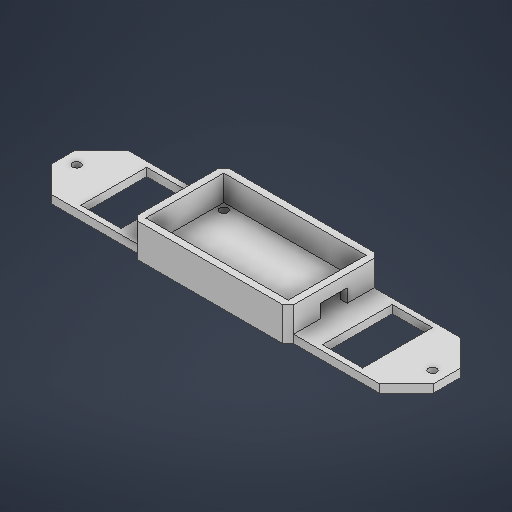
# Autodesk Inventor part: espbase
Saved by Autodesk Inventor 2026 (Build 300175050, 175E)
## iProperties
Created: 2025-04-01
Part Number: espbase
Material: Genérico
Document SubType Name: Modeling
Designer: Ian
Density: 1 g/cm^3
Appearance: Padrão
Author: Ian
Autodesk Inventor part; units mm, degrees
ref_plane "YZ Plane" through (0, 0, 0) normal (1, 0, 0) x (0, 1, 0)
ref_plane "XZ Plane" through (0, 0, 0) normal (0, 1, 0) x (-1, 0, 0)
ref_plane "XY Plane" through (0, 0, 0) normal (0, 0, 1) x (1, 0, 0)
sketch "Esboço1" plane through (0, 0, 0) normal (0, 1, 0) x (-1, 0, 0)
  line L0 (-29, 17) -> (29, 17)
  line L1 (29, 17) -> (29, -17)
  line L2 (29, -17) -> (-29, -17)
  line L3 (-29, -17) -> (-29, 17)
  line L4 (-29, 17) -> (29, -17) construction
  line L5 (29, 17) -> (-29, -17) construction
  point P0 (0, 0)
  point P1 (0.0565, -0.0161)
  dimension "d0" = 58
  dimension "d1" = 34
  constraints: 12 end point, 2 midpoint, 2 parallel, 1 horizontal, 1 perpendicular
  measures "d0" distance of L1.end L2.end
  measures "d1" distance of L0.end L1.end
extrude "Extrusão1" add sketch "Esboço1" along normal blind 3
sketch "Esboço2" plane through (0, 3, 0) normal (0, 1, 0) x (1, 0, 0)
  line L0 (26.5, -14.5) -> (-26.5, -14.5)
  line L1 (-26.5, -14.5) -> (-26.5, 14.5)
  line L2 (-26.5, 14.5) -> (26.5, 14.5)
  line L3 (26.5, 14.5) -> (26.5, -14.5)
  line L4 (26.5, -14.5) -> (-26.5, 14.5) construction
  line L5 (-26.5, -14.5) -> (26.5, 14.5) construction
  line L6 (29, 17) -> (-29, 17) projected
  line L7 (29, -17) -> (-29, -17)
  line L8 (-29, -17) -> (-29, 17)
  line L9 (-29, 17) -> (29, 17)
  line L10 (29, 17) -> (29, -17)
  line L11 (29, -17) -> (-29, 17) construction
  line L12 (-29, -17) -> (29, 17) construction
  point P0 (0, 0)
  dimension "d4" = 53
  dimension "d5" = 29
  constraints: 24 end point, 4 midpoint, 4 parallel, 2 horizontal, 2 perpendicular
  measures "d4" distance of L1.end L2.end
  measures "d5" distance of L0.end L1.end
extrude "Extrusão2" add sketch "Esboço2" along normal blind 9.5
sketch "Esboço3" plane through (0, 3, 0) normal (0, 1, 0) x (1, 0, 0)
  circle A0 centre (-24, 12) radius 1.5
  line L0 (-26.5, 14.5) -> (26.5, 14.5) projected
  line L1 (-26.5, -14.5) -> (-26.5, 14.5) projected
  circle A1 centre (24, 12) radius 1.5
  line L2 (26.5, 14.5) -> (26.5, -14.5) projected
  circle A2 centre (-24, -12) radius 1.5
  line L3 (26.5, -14.5) -> (-26.5, -14.5) projected
  circle A3 centre (24, -12) radius 1.5
  point P0 (0, 0)
  point P1 (-13.75, -16.75)
  point P2 (-13.75, 16.75)
  point P3 (13.75, 16.75)
  point P4 (13.75, -16.75)
  dimension "d8" = 3
  dimension "d9" = 2.5
  dimension "d10" = 2.5
  dimension "d11" = 3
  dimension "d12" = 2.5
  dimension "d13" = 2.5
  dimension "d14" = 3
  dimension "d15" = 2.5
  dimension "d16" = 2.5
  dimension "d17" = 3
  dimension "d18" = 2.5
  dimension "d19" = 2.5
  constraints: 4 centre point, 2 other
  measures "d8" diameter of A0
  measures "d9" distance from line of L0 A0.centre
  measures "d11" diameter of A1
  measures "d13" distance from line of L0 A1.centre
  measures "d14" diameter of A2
  measures "d15" distance from line of L3 A2.centre
  measures "d17" diameter of A3
  measures "d19" distance from line of L3 A3.centre
extrude "Extrusão3" cut sketch "Esboço3" against normal through all contours A0 | A1 | A2 | A3
chamfer "Chanfro1" distance 2 angle 45 4 edges at (29, 6.25, 17) (-29, 6.25, 17) (-29, 6.25, -17) (29, 6.25, -17)
sketch "Esboço7" plane through (29, 0, 15) normal (1, 0, 0) x (0, 0, -1)
  line L0 (30, 0) -> (0, 0) projected
  line L1 (0, 0) -> (30, 0)
  line L2 (30, 0) -> (30, 3)
  line L3 (30, 3) -> (0, 3)
  line L4 (0, 3) -> (0, 0)
  line L5 (30, 12.5) -> (30, 0) projected
  line L6 (0, 0) -> (0, 12.5) projected
  point P0 (15, 0)
  point P1 (15, 0)
  point P2 (15, 3)
  dimension "d36" = 3
  dimension "d42" = 0
  dimension "d43" = 0
  constraints: 8 end point, 2 midpoint, 2 parallel, 1 horizontal, 1 perpendicular, 1 point on line
  measures "d36" distance of L2.end L1.end
  measures "d42" horizontal distance of point (15, 0) point (15, 3)
  measures "d43" distance between parallel lines of L6 L4
extrude "Extrusão6" add sketch "Esboço7" along normal blind 42.04
sketch "Esboço9" plane through (-29, 0, -15) normal (-1, 0, 0) x (0, 0, 1)
  line L0 (30, 12.5) -> (30, 0) projected
  line L1 (1.5, 0) -> (30, 0)
  line L2 (30, 0) -> (30, 3)
  line L3 (30, 3) -> (1.5, 3)
  line L4 (1.5, 3) -> (1.5, 0)
  point P0 (15, 0)
  dimension "d59" = 3
  constraints: 8 end point, 2 parallel, 1 horizontal, 1 perpendicular, 1 point on line
  measures "d59" distance of L2.end L1.end
extrude "Extrusão8" add sketch "Esboço9" along normal blind 42.04
sketch "Esboço8" plane through (29, 3, 15) normal (0, 1, 0) x (1, 0, 0)
  circle A0 centre (37.5465, 14.25) radius 1.5
  line L0 (0, 0) -> (0, 30) projected
  line L1 (23.7495, 2) -> (8.7495, 2)
  line L2 (8.7495, 2) -> (8.7495, 28)
  line L3 (8.7495, 28) -> (23.7495, 28)
  line L4 (23.7495, 28) -> (23.7495, 2)
  line L5 (0, 0) -> (42.04, 0) projected
  line L6 (0, 30) -> (42.04, 30) projected
  line L7 (-2, 32) -> (-56, 32) projected
  line L8 (-56, -2) -> (-2, -2) projected
  circle A1 centre (-95.0465, 14.25) radius 1.5
  line L9 (-81.2495, 2) -> (-66.2495, 2)
  line L10 (-66.2495, 2) -> (-66.2495, 26.5)
  line L11 (-66.2495, 26.5) -> (-81.2495, 26.5)
  line L12 (-81.2495, 26.5) -> (-81.2495, 2)
  point P0 (-29, 15)
  point P1 (23.7495, 15)
  point P2 (-81.2495, 14.25)
  dimension "d44" = 3
  dimension "d47" = 13.797
  dimension "d53" = 2
  dimension "d54" = 2
  dimension "d55" = 15
  constraints: 16 end point, 2 centre point, 2 parallel, 1 horizontal, 1 midpoint, 1 perpendicular
  measures "d44" diameter of A0
  measures "d47" horizontal distance of point (23.749, 15) A0.centre
  measures "d53" distance between parallel lines of L5 L1
  measures "d54" distance between parallel lines of L6 L3
  measures "d55" distance between parallel lines of L2 L4
extrude "Extrusão7" cut sketch "Esboço8" against normal blind 42.04
chamfer "Chanfro2" distance 10 angle 45 4 edges at (71.04, 1.5, -15) (71.04, 1.5, 15) (-71.04, 1.5, -13.5) (-71.04, 1.5, 15)
sketch "Esboço10" plane through (29, 12.5, 15) normal (1, 0, 0) x (0, 0, -1)
  line L0 (0, -9.5) -> (30, -9.5) projected
  line L1 (30, 0) -> (30, -9.5) projected
  line L2 (0, 0) -> (30, 0) projected
  line L3 (0, -9.5) -> (0, 0) projected
  line L4 (10, -12.5) -> (10, -9.5) projected
  line L5 (10, -12.5) -> (20, -12.5) projected
  line L6 (20, -9.5) -> (20, -12.5) projected
  line L7 (20, -9.5) -> (10, -9.5) projected
  line L8 (10, -9.5) -> (20, -9.5)
  line L9 (20, -9.5) -> (20, -4.5)
  line L10 (20, -4.5) -> (10, -4.5)
  line L11 (10, -4.5) -> (10, -9.5)
  point P0 (15, -12.5)
  dimension "d63" = 5
  constraints: 8 end point, 2 parallel, 1 horizontal, 1 perpendicular
  measures "d63" distance of L9.end L8.end
extrude "Extrusão9" cut sketch "Esboço10" against normal blind 10 contours L11 L10 L9 L0
